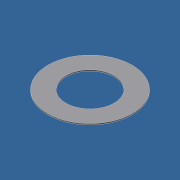
# Autodesk Inventor part: BN1976-8x14x0.2
Saved by Autodesk Inventor 2021.3 (Build 253353000, 353)
## iProperties
Created: 2023-01-19
Part Number: BN1976-8x14x0.2
Project: Visserie
Material: .115CrV3/K510
Description: Rondelle d'ajustage
Document SubType Name: Modeling
Designer: Jean-Marc.VULLIAMY
Authority: DIN 988
Mass: 0.0924806 g
Surface Area: 1.27235 cm^2
Volume: 0.011781 cm^3
Density: 7.85 g/cm^3
Appearance: Par défaut
Material number: ---
Author: Jean-Marc.VULLIAMY
Autodesk Inventor part; units mm, degrees
ref_plane "Plan YZ" through (0, 0, 0) normal (1, 0, 0) x (0, 1, 0)
ref_plane "Plan XZ" through (0, 0, 0) normal (0, 1, 0) x (-1, 0, 0)
ref_plane "Plan XY" through (0, 0, 0) normal (0, 0, 1) x (1, 0, 0)
sketch "Esquisse1" plane through (0, 0, 0) normal (0, 0, 1) x (1, 0, 0)
  circle A0 centre (0, 0) radius 4
  circle A1 centre (0, 0) radius 7
  dimension "d0" = 8
  dimension "d1" = 14
  constraints: 2 centre point, 2 coincident
  measures "d0" diameter of A0
  measures "d1" diameter of A1
extrude "Extrusion1" add sketch "Esquisse1" along normal blind 0.2
